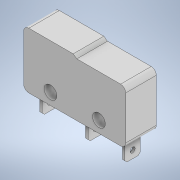
# Autodesk Inventor part: limitSwitch
Saved by Autodesk Inventor 2020.2 (Build 242310000, 310)
## iProperties
Created: 2020-04-12
Part Number: limitSwitch
Material: Generic
Document SubType Name: Modeling
Designer: Josiah
Density: 1 g/cm^3
Appearance: Default
Author: Josiah
Autodesk Inventor part; units mm, degrees
ref_plane "YZ Plane" through (0, 0, 0) normal (1, 0, 0) x (0, 1, 0)
ref_plane "XZ Plane" through (0, 0, 0) normal (0, 1, 0) x (-1, 0, 0)
ref_plane "XY Plane" through (0, 0, 0) normal (0, 0, 1) x (1, 0, 0)
sketch "Sketch1" plane through (0, 0, 0) normal (0, 0, 1) x (1, 0, 0)
  line L0 (-10, 5.5) -> (-0.289, 5.5)
  line L1 (10, 5) -> (10, -5.5)
  line L2 (10, -5.5) -> (-10, -5.5)
  line L3 (-10, -5.5) -> (-10, 5.5)
  line L4 (-0.289, 5.5) -> (0.4244, 5)
  line L5 (0.4244, 5) -> (10, 5)
  line L6 (-10, 5.5) -> (10, -5.5) construction
  circle A0 centre (4.75, -3.25) radius 1.25
  line L7 (0, -5.5) -> (0, 3.5475) construction
  circle A1 centre (-4.75, -3.25) radius 1.25
  point P0 (0, 0)
  point P1 (0, 0)
  point P2 (0, 0)
  dimension "d3" = 20
  dimension "d4" = 11
  dimension "d5" = 10.5
  dimension "d6" = 0.7134
  dimension "d7" = 2.5
  dimension "d8" = 2.25
  dimension "d9" = 5.25
  constraints: 17 end point, 2 centre point, 2 coincident, 2 midpoint, 2 parallel, 2 perpendicular, 1 horizontal, 1 symmetric about line, 1 vertical, 1 other
  measures "d3" distance of L1.end L2.end
  measures "d4" distance between parallel lines of L0 L2
  measures "d5" distance of L1.start L1.end
  measures "d6" horizontal distance of L0.end L4.end
  measures "d7" diameter of A0
  measures "d8" distance from line of L2 A0.centre
  measures "d9" distance from line of L1 A0.centre
extrude "Extrusion1" add sketch "Sketch1" along normal blind 6
sketch "Sketch2" plane through (-10, -5.5, 0) normal (0, -1, 0) x (1, 0, 0)
  line L0 (1.65, 4.5) -> (2.15, 4.5)
  line L1 (2.15, 4.5) -> (2.15, 1.5)
  line L2 (2.15, 1.5) -> (1.65, 1.5)
  line L3 (1.65, 1.5) -> (1.65, 4.5)
  line L4 (10.65, 4.5) -> (11.15, 4.5)
  line L5 (11.15, 4.5) -> (11.15, 1.5)
  line L6 (11.15, 1.5) -> (10.65, 1.5)
  line L7 (10.65, 1.5) -> (10.65, 4.5)
  line L8 (17.85, 4.5) -> (18.35, 4.5)
  line L9 (18.35, 4.5) -> (18.35, 1.5)
  line L10 (18.35, 1.5) -> (17.85, 1.5)
  line L11 (17.85, 1.5) -> (17.85, 4.5)
  line L12 (0, 0) -> (0, 6) projected
  line L13 (0, 0) -> (20, 0) projected
  line L14 (0, 6) -> (20, 6) projected
  point P0 (10, 0)
  dimension "d12" = 3
  dimension "d13" = 3
  dimension "d14" = 3
  dimension "d15" = 0.5
  dimension "d16" = 0.5
  dimension "d17" = 0.5
  dimension "d18" = 1.65
  dimension "d19" = 8.5
  dimension "d20" = 6.7
  dimension "d21" = 6
  dimension "d22" = 1.5
  constraints: 24 end point, 6 parallel, 3 horizontal, 3 perpendicular, 2 point on line
  measures "d12" distance of L0.end L1.end
  measures "d13" distance of L4.end L5.end
  measures "d14" distance of L10.end L8.start
  measures "d15" distance of L0.start L0.end
  measures "d16" distance of L4.start L4.end
  measures "d17" distance of L8.start L8.end
  measures "d18" distance between parallel lines of L12 L3
  measures "d19" distance between parallel lines of L7 L1
  measures "d20" distance between parallel lines of L11 L5
  measures "d21" distance between parallel lines of L13 L14
  measures "d22" distance between parallel lines of L14 L0
extrude "Extrusion2" add sketch "Sketch2" along normal blind 4
sketch "Sketch3" plane through (8.35, -5.5, 4.5) normal (1, 0, 0) x (0, 0, -1)
  circle A0 centre (1.5, -2.5) radius 0.5
  line L0 (3, -4) -> (0, -4) projected
  line L1 (3, 0) -> (3, -4) projected
  line L2 (0, 0) -> (0, -4) projected
  point P0 (4.5, 5.5)
  dimension "d25" = 1
  dimension "d26" = 1.5
  dimension "d27" = 3
  dimension "d28" = 1.5
  constraints: 1 centre point
  measures "d25" diameter of A0
  measures "d26" distance from line of L0 A0.centre
  measures "d27" distance between parallel lines of L1 L2
  measures "d28" distance from line of A0.centre L2
extrude "Extrusion3" cut sketch "Sketch3" against normal through all
chamfer "Chamfer1" distance 0.4 angle 45 6 edges at (8.1, -9.5, 4.5) (8.1, -9.5, 1.5) (0.9, -9.5, 1.5) (0.9, -9.5, 4.5) (-8.1, -9.5, 4.5) (-8.1, -9.5, 1.5)
fillet "Fillet1" radius 1 4 edges at (10, 5, 3) (10, -5.5, 3) (-10, -5.5, 3) (-10, 5.5, 3)
equation "\"d13\" = d12"
equation "\"d14\" = d13"
equation "\"d22\" = -0.5 * d12 + 0.5 * d21"
equation "\"d28\" = 0.5 * d27"
body "Solid1"
